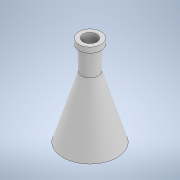
# Autodesk Inventor part: Модель колба коническая 25мл
Saved by Autodesk Inventor 2022 (Build 260153000, 153)
## iProperties
Created: 2022-06-09
Part Number: Модель колба коническая 25мл
Material: Типовые
Document SubType Name: Modeling
Designer: Admin
Density: 1 g/cm^3
Appearance: По умолчанию
Author: Admin
Autodesk Inventor part; units mm, degrees
ref_plane "YZ Plane" through (0, 0, 0) normal (1, 0, 0) x (0, 1, 0)
ref_plane "XZ Plane" through (0, 0, 0) normal (0, 1, 0) x (-1, 0, 0)
ref_plane "XY Plane" through (0, 0, 0) normal (0, 0, 1) x (1, 0, 0)
sketch "Эскиз1" plane through (0, 0, 0) normal (0, 0, 1) x (1, 0, 0)
  line L0 (0, 0) -> (25.5, 0)
  line L1 (25.5, 0) -> (8, 58)
  line L2 (8, 58) -> (8.4582, 79)
  line L3 (10.5, 80) -> (10.5, 85)
  line L4 (10.5, 85) -> (6.5, 85)
  line L5 (6.5, 85) -> (5.9109, 58)
  line L6 (5.9109, 58) -> (22.8075, 2)
  line L7 (22.8075, 2) -> (0, 2)
  line L8 (0, 21.2466) -> (0, -2.9394)
  line L9 (8.4582, 79) -> (10.5, 80)
  point P0 (0, 2)
  dimension "d0" = 51
  dimension "d1" = 2
  dimension "d2" = 2
  dimension "d3" = 58
  dimension "d4" = 85
  dimension "d5" = 5
  dimension "d6" = 16
  dimension "d8" = 21
  dimension "d9" = 4
  dimension "d10" = 21
  constraints: 20 end point, 3 parallel, 2 horizontal, 1 horizontal alignment, 1 perpendicular, 1 vertical, 1 vertical alignment
  measures "d0" diameter of L0.end L8
  measures "d1" distance between parallel lines of L7 L0
  measures "d2" distance between parallel lines of L1 L6
  measures "d3" vertical distance of L1.end L0.end
  measures "d4" distance between parallel lines of L4 L0
  measures "d5" distance of L3.start L3.end
  measures "d6" diameter of L1.end L8
  measures "d8" diameter of L3 L8
  measures "d9" distance of L3.end L4.end
  measures "d10" vertical distance of L2.end L1.end
revolve "Вращение1" add sketch "Эскиз1" angle 360 about axis through (0, 21.2466, 0) along (0, -1, 0)
